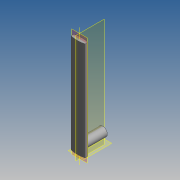
# Autodesk Inventor part: P032_Antenne
Saved by Autodesk Inventor 2021.3 (Build 253353000, 353)
## iProperties
Created: 2021-11-26
Part Number: P032_Antenne
Material: Générique
Document SubType Name: Modeling
Designer: gabri
Density: 1 g/cm^3
Appearance: Par défaut
Author: gabri
Autodesk Inventor part; units mm, degrees
sketch "Sketch2" plane through (0, 0, 0) normal (0, 0, 1) x (1, 0, 0)
  line L0 (10, -2) -> (-10, -2)
  line L1 (-10, -2) -> (-10, 2)
  line L2 (-10, 2) -> (10, 2)
  line L3 (10, 2) -> (10, -2)
  line L4 (10, -2) -> (-10, 2) construction
  line L5 (-10, -2) -> (10, 2) construction
  arc A0 (10, 2) -> (-10, 2) centre (0, -36.7298) ccw
  arc A1 (-10, -2) -> (10, -2) centre (0, 36.7298) ccw
  point P0 (0, 0)
  dimension "d0" = 20
  dimension "d1" = 4
  dimension "d2" = 40
  dimension "d3" = 40
  constraints: 12 end point, 4 point on circle, 2 centre point, 2 midpoint, 2 parallel, 1 horizontal, 1 perpendicular
  measures "d0" distance of L1.end L2.end
  measures "d1" distance between parallel lines of L0 L2
  measures "d2" radius of A0
  measures "d3" radius of A1
extrude "Extrusion1" add sketch "Sketch2" along normal blind 140
sketch "Sketch3" plane through (0, 0, 0) normal (0, 1, 0) x (-1, 0, 0)
  circle A0 centre (0, 10) radius 6.5
  line L0 (0, -28) -> (0, 168) construction
  line L1 (14, 0) -> (-14, 0) construction
  point P0 (0, 0)
  dimension "d6" = 13
  dimension "d7" = 10
  constraints: 1 centre point, 1 point on line
  measures "d6" diameter of A0
  measures "d7" distance from line of L1 A0.centre
extrude "Extrusion2" add sketch "Sketch3" along normal blind 33
body "Solid1"
